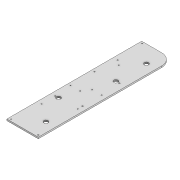
# Autodesk Inventor part: sidewall outside
Saved by Autodesk Inventor 2020 (Build 240168000, 168)
## iProperties
Created: 2020-03-01
Part Number: sidewall outside
Material: Generic
Document SubType Name: Modeling
Designer: ball
Density: 1 g/cm^3
Appearance: Default
Author: ball
Autodesk Inventor part; units mm, degrees
ref_plane "YZ Plane" through (0, 0, 0) normal (1, 0, 0) x (0, 1, 0)
ref_plane "XZ Plane" through (0, 0, 0) normal (0, 1, 0) x (-1, 0, 0)
ref_plane "XY Plane" through (0, 0, 0) normal (0, 0, 1) x (1, 0, 0)
sketch "Sketch1" plane through (0, 0, 0) normal (0, 1, 0) x (-1, 0, 0)
  line L0 (0, 0) -> (104.9602, 0)
  line L1 (104.9602, 0) -> (104.9602, -450.85)
  line L2 (104.9602, -450.85) -> (38.1, -450.85)
  line L3 (0, -412.75) -> (0, 0)
  arc A0 (0, -412.75) -> (38.1, -450.85) centre (38.1, -412.75) ccw
  line L4 (38.1, -412.75) -> (38.1, -450.85) construction
  line L5 (38.1, -412.75) -> (76.2, -412.75) construction
  dimension "d1" = 450.85
  dimension "d5" = 38.1
  dimension "d6" = 90
  dimension "d7" = 104.9602
  dimension "d8" = 38.1
  constraints: 12 end point, 2 horizontal, 2 parallel, 2 perpendicular, 2 point on circle, 1 centre point, 1 coincident
  measures "d1" distance of L0.end L1.end
  measures "d5" radius of A0
  measures "d6" angle of L4 L5
  measures "d7" distance between parallel lines of L3 L1
  measures "d8" distance from line of L3 point (38.1, -412.75)
extrude "Extrusion1" add sketch "Sketch1" along normal blind 5
sketch "Sketch2" plane through (0, 5, 0) normal (0, 1, 0) x (1, 0, 0)
  circle A0 centre (-31.75, 57.3786) radius 7.1016
  line L0 (-104.9602, 0) -> (0, 0) projected
  line L1 (0, 0) -> (0, 412.75) projected
  circle A1 centre (-31.75, 393.4714) radius 7.1016
  circle A2 centre (-6.35, 6.35) radius 2.25
  dimension "BearingHole" = 14.2032
  dimension "d12" = 57.3786
  dimension "d13" = 31.75
  dimension "d14" = 14.2032
  dimension "d15" = 31.75
  dimension "d16" = 336.0928
  dimension "M4Clearance" = 4.5
  dimension "d71" = 6.35
  dimension "d72" = 6.35
  constraints: 3 centre point
  measures "BearingHole" diameter of A0
  measures "d12" distance from line of L0 A0.centre
  measures "d13" distance from line of L1 A0.centre
  measures "d14" diameter of A1
  measures "d15" distance from line of L1 A1.centre
  measures "d16" distance of A0.centre A1.centre
  measures "M4Clearance" diameter of A2
  measures "d71" distance from line of L1 A2.centre
  measures "d72" distance from line of L0 A2.centre
extrude "Extrusion2" cut sketch "Sketch2" against normal through all
sketch "Sketch3" plane through (0, 5, 0) normal (0, 1, 0) x (1, 0, 0)
  circle A0 centre (-97.3271, 444.4951) radius 1.7 construction
  circle A1 centre (-97.3271, 6.3451) radius 1.7 construction
  circle A2 centre (-63.6771, 179.4396) radius 3.15 construction
  circle A3 centre (-95.6771, 179.4396) radius 3.5 construction
  circle A4 centre (-79.6771, 147.4247) radius 7 construction
  circle A5 centre (-31.6771, 291.4544) radius 7 construction
  circle A6 centre (-15.6771, 259.4396) radius 3.5 construction
  circle A7 centre (-47.6771, 259.4396) radius 3.5 construction
  circle A8 centre (-31.75, 393.4714) radius 7.1016 construction
  circle A9 centre (-15.6771, 163.4396) radius 2.25 construction
  arc A10 (-33.6771, 302.7533) -> (-29.6771, 302.7533) centre (-31.6771, 302.7533) ccw construction
  arc A11 (-29.6771, 304.1259) -> (-33.6771, 304.1259) centre (-31.6771, 304.1259) ccw construction
  line L0 (-29.6771, 302.7533) -> (-29.6771, 304.1259) construction
  line L1 (-33.6771, 304.1259) -> (-33.6771, 302.7533) construction
  line L2 (-77.6771, 158.7533) -> (-77.6771, 160.1259) construction
  arc A12 (-77.6771, 160.1259) -> (-81.6771, 160.1259) centre (-79.6771, 160.1259) ccw construction
  line L3 (-81.6771, 160.1259) -> (-81.6771, 158.7533) construction
  arc A13 (-81.6771, 158.7533) -> (-77.6771, 158.7533) centre (-79.6771, 158.7533) ccw construction
  circle A14 centre (-97.3271, 6.3451) radius 1.7
  circle A15 centre (-97.3271, 444.4951) radius 1.7
  circle A16 centre (-79.6771, 147.4247) radius 7.1016
  circle A17 centre (-31.6771, 291.4544) radius 7.1016
  circle A18 centre (-15.6771, 163.4396) radius 2.286
  arc A19 (-77.6771, 136.1259) -> (-81.6771, 136.1259) centre (-79.6771, 136.1259) ccw construction
  line L4 (-77.6771, 134.7533) -> (-77.6771, 136.1259) construction
  line L5 (-81.6771, 136.1259) -> (-81.6771, 134.7533) construction
  arc A20 (-81.6771, 134.7533) -> (-77.6771, 134.7533) centre (-79.6771, 134.7533) ccw construction
  circle A21 centre (-90.4602, 355.95) radius 1.7 construction
  circle A22 centre (-90.4602, 355.95) radius 1.7
  circle A23 centre (-90.4602, 101.631) radius 1.7 construction
  circle A24 centre (-90.4602, 101.631) radius 1.7
  point P0 (0, 0)
  dimension "d75" = 3.4
  dimension "d76" = 3.4
  dimension "BearingClearance" = 14.2032
  dimension "d78" = 14.2032
  dimension "d83" = 4.572
  dimension "d90" = 3.4
  dimension "d91" = 3.4
  constraints: 7 centre point, 7 coincident
  measures "d75" diameter of A14
  measures "d76" diameter of A15
  measures "BearingClearance" diameter of A16
  measures "d78" diameter of A17
  measures "d83" diameter of A18
  measures "d90" diameter of A22
  measures "d91" diameter of A24
extrude "Extrusion3" cut sketch "Sketch3" against normal through all
sketch "Sketch4" plane through (0, 0, 0) normal (0, -1, 0) x (1, 0, 0)
  circle A0 centre (-73.66, -342.9) radius 1.7 construction
  circle A1 centre (-95.6771, -203.4396) radius 1.9304 construction
  circle A2 centre (-47.6771, -227.4396) radius 1.9304 construction
  circle A3 centre (-15.6771, -227.4396) radius 1.9304 construction
  circle A4 centre (-54.3045, -291.4544) radius 2 construction
  circle A5 centre (-95.6771, -283.4396) radius 1.9304 construction
  circle A6 centre (-63.6771, -203.4396) radius 1.9304 construction
  circle A7 centre (-63.6771, -203.4396) radius 1.9304 construction
  circle A8 centre (-15.6771, -147.4396) radius 1.9304 construction
  circle A9 centre (-73.66, -342.9) radius 1.7
  circle A10 centre (-95.6771, -283.4396) radius 1.7
  circle A11 centre (-47.6771, -227.4396) radius 1.7
  circle A12 centre (-15.6771, -227.4396) radius 1.7
  circle A13 centre (-95.6771, -203.4396) radius 1.7
  circle A14 centre (-63.6771, -203.4396) radius 1.7
  circle A15 centre (-15.6771, -147.4396) radius 1.7
  point P0 (0, 0)
  dimension "d92" = 3.4
  dimension "d93" = 3.4
  dimension "d94" = 3.4
  dimension "d95" = 3.4
  dimension "d96" = 3.4
  dimension "d97" = 3.4
  dimension "d98" = 3.4
  constraints: 7 centre point, 7 coincident
  measures "d92" diameter of A9
  measures "d93" diameter of A10
  measures "d94" diameter of A11
  measures "d95" diameter of A12
  measures "d96" diameter of A13
  measures "d97" diameter of A14
  measures "d98" diameter of A15
extrude "Extrusion4" cut sketch "Sketch4" against normal through all
sketch "Sketch5" plane through (0, 0, 0) normal (0, -1, 0) x (1, 0, 0)
  circle A0 centre (-90.9801, -147.4247) radius 2
  circle A1 centre (-79.6771, -147.4247) radius 7.1016 projected
  circle A2 centre (-20.3741, -291.4544) radius 2
  circle A3 centre (-31.6771, -291.4544) radius 7.1016 projected
  point P0 (0, 0)
  dimension "d101" = 4
  dimension "d102" = 11.303
  dimension "d103" = 4
  dimension "d104" = 11.303
  constraints: 2 centre point
  measures "d101" diameter of A0
  measures "d102" distance of A0.centre A1.centre
  measures "d103" diameter of A2
  measures "d104" distance of A2.centre A3.centre
extrude "Extrusion5" cut sketch "Sketch5" against normal through all contours A0 | A2
equation "\"d14\" = BearingHole"
equation "\"d15\" = d13"
equation "\"d75\" = M3Clearance"
equation "\"d76\" = M3Clearance"
equation "\"BearingClearance\" = BearingHole"
equation "\"d78\" = BearingHole"
equation "\"d90\" = M3Clearance"
equation "\"d91\" = M3Clearance"
equation "\"d92\" = M3Clearance"
equation "\"d93\" = M3Clearance"
equation "\"d94\" = M3Clearance"
equation "\"d95\" = M3Clearance"
equation "\"d96\" = M3Clearance"
equation "\"d97\" = M3Clearance"
equation "\"d98\" = M3Clearance"
equation "\"d103\" = d101"
equation "\"d104\" = d102"
equation "\"M3Clearance\" = 3.4"
body "Solid1"
